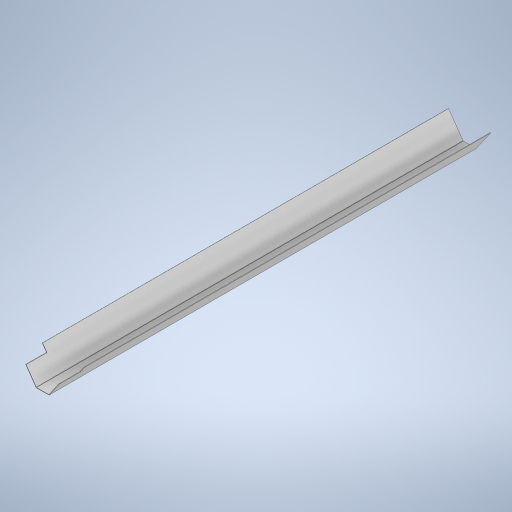
# Autodesk Inventor part: ДМС 040 лоток илоотвод
Saved by Autodesk Inventor 2024.2 (Build 282272000, 272)
## iProperties
Created: 2023-09-04
Part Number: ДМС 040 лоток илоотвод
Material: Generic
Document SubType Name: Sheet Metal
Designer: admin
Density: 1 g/cm^3
Sheet Metal Rule: Default_mm
Appearance: Default
Лоток_ширина_низ: 60,000 mm
Лоток_ширина_верх: 200,000 mm
Лоток_высота: 100,000 mm
Лоток_угол: 125,00 deg
Лоток_глубина_выреза: 30,000 mm
Author: admin
Autodesk Inventor part; units mm, degrees
ref_plane "YZ Plane" through (0, 0, 0) normal (1, 0, 0) x (0, 1, 0)
ref_plane "XZ Plane" through (0, 0, 0) normal (0, 1, 0) x (-1, 0, 0)
ref_plane "XY Plane" through (0, 0, 0) normal (0, 0, 1) x (1, 0, 0)
sketch "Sketch4" plane through (0, 0, 0) normal (0, 0, 1) x (1, 0, 0)
  line L0 (-30, 0) -> (-28.9589, 0) construction
  line L1 (30, 0) -> (30.5972, 0.8528) construction
  line L2 (-30, 0) -> (-30.5972, 0.8528) construction
  line L3 (-100.0208, 100) -> (100.0208, 100) construction
  arc A0 (-30.5972, 0.8528) -> (-28.9589, 0) centre (-28.9589, 2) ccw
  arc A1 (28.9589, 0) -> (30.5972, 0.8528) centre (28.9589, 2) ccw
  line L4 (28.9589, 0) -> (30, 0) construction
  line L5 (30.5972, 0.8528) -> (100.0208, 100)
  line L6 (-30.5972, 0.8528) -> (-100.0208, 100)
  line L7 (-28.9589, 0) -> (28.9589, 0)
  point P0 (0, 0)
  point P1 (0, 0)
  point P2 (0, 100)
  point P3 (0, 0)
  dimension "d14" = 200.0415
  dimension "d15" = 60
  dimension "d16" = 100
  dimension "d17" = 2
  dimension "d39" = 125
  measures "d14" distance of L3.start L3.end
  measures "d15" distance of L0.start L1.start
  measures "d16" distance between parallel lines of L0 L3
  measures "d17" radius of A0
  measures "d39" angle of L7 L6
contour flange "Contour Flange2" sketch "Sketch4" thickness 2 bend radius 2 width 2050 along (0, 0, -1) mid plane no both sides no wall seen from (-65.309, 50.4264, 0) lies toward (-0.819152, -0.5735764, 0) curves L6 A0 L7 A1 L5
bend "Bend4"
corner "Corner4"
sketch "Sketch6" plane through (0, 0, 0) normal (1, 0, 0) x (0, 1, 0)
  line L0 (100, -2050) -> (100, 0) projected
  line L1 (-0.2943, 0) -> (98.8528, 0) projected
  line L2 (98.8528, 0) -> (98.8528, -2050) projected
  line L3 (98.8528, 0) -> (100, 0)
  line L4 (70, 0) -> (70, -100)
  line L5 (70, -100) -> (100, -100)
  point P0 (0, 0)
  dimension "d51" = 30
  dimension "d52" = 100
  constraints: 6 end point, 2 perpendicular, 2 point on line, 1 vertical
  measures "d51" distance of L4.end L5.end
  measures "d52" distance of L4.start L4.end
extrude "Extrusion1" cut sketch "Sketch6" along normal through all both and the other way through all
equation "\"d17\" = BendRadius"
equation "\"d51\" = Лоток_глубина_выреза"
equation "\"d40\" = Thickness"
equation "\"d41\" = BendReliefWidth"
equation "\"d42\" = BendReliefDepth"
equation "\"d43\" = MinimumRemnant"
equation "\"d44\" = TransitionRadius"
equation "\"d46\" = BendRadius"
equation "\"d48\" = CornerReliefSize"
equation "\"d49\" = GapSize"
equation "\"d50\" = JacobiRadiusSize"
equation "\"BendRadius\" = Thickness"
equation "\"BendReliefWidth\" = Thickness"
equation "\"BendReliefDepth\" = 0.5 * Thickness"
equation "\"CornerReliefSize\" = 4 * Thickness"
equation "\"MinimumRemnant\" = 2 * Thickness"
equation "\"TransitionRadius\" = BendRadius"
equation "\"JacobiRadiusSize\" = BendRadius"
equation "\"GapSize\" = Thickness"
equation "\"Лоток_ширина_низ\" = 60"
equation "\"Лоток_ширина_верх\" = 200"
equation "\"Лоток_высота\" = 100"
equation "\"Лоток_угол\" = 125deg"
equation "\"Лоток_глубина_выреза\" = 30"
equation "\"Thickness\" = 2"
body "Solid3"
